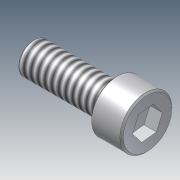
# Autodesk Inventor part: HW-00070
Saved by Autodesk Inventor 2012 (Build 160160000, 160)
## iProperties
Created: 2008-05-28
Part Number: HW-00070
Document SubType Name: Modeling
Designer: mcyr
Density: 1 g/cm^3
Description: Hex SHCS, 10-24 x .5"
Material: Default
Title: Hex SHCS, 10-24 x .5"
Author: mcyr
Autodesk Inventor part; units mm, degrees
ref_plane "YZ Plane" through (0, 0, 0) normal (1, 0, 0) x (0, 1, 0)
ref_plane "XZ Plane" through (0, 0, 0) normal (0, 1, 0) x (-1, 0, 0)
ref_plane "XY Plane" through (0, 0, 0) normal (0, 0, 1) x (1, 0, 0)
sketch "Sketch1" plane through (0, 0, 0) normal (0, 0, 1) x (1, 0, 0)
  line L0 (-20.0958, 2.2922) -> (-2.5698, 2.2922)
  line L1 (-2.5698, 2.2922) -> (-2.5698, 6.2546)
  line L2 (-2.5698, 6.2546) -> (-7.3958, 6.2546)
  line L3 (-7.3958, 6.2546) -> (-7.3958, 4.6798)
  line L4 (-7.3958, 4.6798) -> (-20.0958, 4.6798)
  line L5 (-20.0958, 4.6798) -> (-20.0958, 2.2922)
  dimension "d0" = 12.7
  dimension "d1" = 2.3876
  dimension "d2" = 4.826
  dimension "d3" = 3.9624
  constraints: 12 end point, 4 parallel, 1 horizontal, 1 perpendicular
  measures "d0" distance of L3.end L4.end
  measures "d1" distance of L4.end L0.start
  measures "d2" distance of L1.end L2.end
  measures "d3" distance of L0.end L1.end
revolve "Revolution1" add sketch "Sketch1" angle 360 about axis through (-20.0958, 2.2922, 0) along (1, 0, 0)
thread "Thread1" size "10-24 UNC" class "2A" standard "ANSI Unified Screw Threads" full length
sketch "Sketch2" plane through (-2.5698, 2.2922, 0) normal (1, 0, 0) x (0, 0, -1)
  circle A0 centre (0, 0) radius 3.9624 projected
  line L0 (-1.3654, 1.8401) -> (0.9109, 2.1025)
  line L1 (0.9109, 2.1025) -> (2.2763, 0.2624)
  line L2 (2.2763, 0.2624) -> (1.3654, -1.8401)
  line L3 (1.3654, -1.8401) -> (-0.9109, -2.1025)
  line L4 (-0.9109, -2.1025) -> (-2.2763, -0.2624)
  line L5 (-2.2763, -0.2624) -> (-1.3654, 1.8401)
  dimension "d18" = 3.9688
  constraints: 12 end point, 1 coincident, 13 other
  measures "d18" distance between parallel lines of L5 L2
extrude "Extrusion1" cut sketch "Sketch2" against normal blind 1.905 contours L0 L1 L2 L3 L4 L5
chamfer "Chamfer1" distance 0.254 angle 45 3 edges at (-2.5698, -1.6702, 0) (-7.3958, -1.6702, 0) (-20.0958, -0.0954, 0)
body "Solid1"
